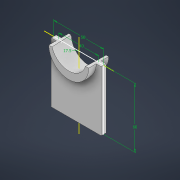
# Autodesk Inventor part: 零件1
Saved by Autodesk Inventor 2021 (Build 250183000, 183)
## iProperties
Created: 2020-12-24
Part Number: 零件1
Material: 一般
Document SubType Name: Modeling
Designer: zihon
Density: 1 g/cm^3
Appearance: 預設
Author: zihon
Autodesk Inventor part; units mm, degrees
ref_plane "YZ Plane" through (0, 0, 0) normal (1, 0, 0) x (0, 1, 0)
ref_plane "XZ Plane" through (0, 0, 0) normal (0, 1, 0) x (-1, 0, 0)
ref_plane "XY Plane" through (0, 0, 0) normal (0, 0, 1) x (1, 0, 0)
sketch "草圖1" plane through (0, 0, 0) normal (0, 0, 1) x (1, 0, 0)
  arc A0 (-17.5, 0) -> (17.5, 0) centre (0, 0) ccw
  arc A1 (-20, 0) -> (20, 0) centre (0, 0) ccw
  line L0 (-20, 0) -> (-17.5, 0)
  line L1 (20, 0) -> (17.5, 0)
  line L2 (-35, 0) -> (35, 0) projected
  line L3 (-25, 0) -> (25, 0)
  line L4 (25, -60) -> (-25, -60)
  line L5 (-25, -60) -> (-25, 0)
  line L6 (-25, 0) -> (25, 0)
  line L7 (25, 0) -> (25, -60)
  line L8 (25, -60) -> (-25, 0) construction
  line L9 (-25, -60) -> (25, 0) construction
  line L10 (0, -72) -> (0, 12) projected
  point P0 (17.5, 0)
  point P1 (20, 0)
  point P2 (20, 0)
  point P3 (0, -30)
  dimension "d16" = 50
  dimension "d17" = 60
  dimension "d22" = 40
  dimension "d23" = 17.5
  constraints: 18 end point, 4 point on circle, 3 horizontal, 3 midpoint, 3 point on line, 2 centre point, 2 collinear, 2 parallel, 1 coincident, 1 perpendicular
  measures "d16" distance between parallel lines of L7 L5
  measures "d17" distance between parallel lines of L4 L3
  measures "d22" distance of L1.start L0.start
  measures "d23" radius of A0
extrude "擠出1" add sketch "草圖1" along normal mid plane 20 contours L2 L10 A0 | A0 L10 A1 L0 | L10 L2 A0 | A0 L1 A1 L10
extrude "擠出2" add sketch "草圖1" along normal mid plane 5
sketch "草圖2" plane through (0, 0, 0) normal (1, 0, 0) x (0, 1, 0)
  line L0 (-10, -10) -> (-5, 10)
  line L1 (0, -2.5) -> (0, -10) projected
  line L2 (0, 10) -> (0, 2.5) projected
  line L3 (-20, -10) -> (0, -10) projected
  line L4 (0, 10) -> (-20, 10) projected
  point P0 (0, 0)
  dimension "d18" = 10
  dimension "d19" = 5
  constraints: 2 end point, 1 midpoint, 1 point on line
  measures "d18" distance from line of L1 L0.start
  measures "d19" distance from line of L2 L0.end
sketch "草圖3" plane through (0, 0, -10) normal (0, 0, -1) x (-1, 0, 0)
  arc A0 (-17.5, 0) -> (17.5, 0) centre (0, 0) ccw projected
  line L0 (25, 0) -> (-25, 0) projected
sweep "掃掠1" cut profiles "草圖3" path "草圖2" path curves L0
